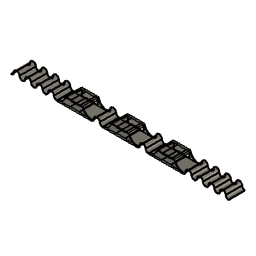
ACUTE_Prototype 4 v1 (Autodesk Fusion 360 design; units mm, degrees)
Autodesk Fusion 360 part; units mm, degrees
note: some values were not read from the file. Chosen so that the rebuilt part matches the saved one: which bodies a step acts on. Set by a fixed rule: which sketch regions a step uses.
sketch "Sketch2" plane through (0, 0, 0) normal (0, 1, 0) x (1, 0, 0)
  line L0 (0, 0) -> (0, -4) construction
  line L1 (0, -4) -> (1, -4) construction
  circle A0 centre (4, -4) radius 4
  circle A1 centre (4, -4) radius 3
  circle A2 centre (11, -4) radius 3
  circle A3 centre (11, -4) radius 4
  circle A4 centre (18, -4) radius 3
  circle A5 centre (18, -4) radius 4
  line L2 (18, 0) -> (18, -1)
  line L3 (18, 0) -> (39, 0)
  line L4 (39, 0) -> (39, -10)
  line L5 (39, -10) -> (18, -10) construction
  line L6 (18, -10) -> (18, 0) construction
  line L7 (28.5, 0) -> (28.5, -10) construction
  line L8 (18, -1) -> (28.5, -1) construction
  arc A6 (28.5, -10) -> (18, -1) centre (18, -11.625) ccw
  line L9 (28.5, -10) -> (39, -10)
  line L10 (4, 0) -> (4, -4)
  line L11 (28.5, 0) -> (29.5, 0) construction
  line L12 (29.5, 0) -> (29.5, -10)
  line L13 (29.5, -10) -> (28.5, -10) construction
  line L14 (28.5, -10) -> (28.5, 0) construction
  line L15 (28.5, -1) -> (29.5, -1) construction
  line L16 (28.5, -1) -> (29.5, -1) construction
  line L17 (29.5, -1) -> (29.5, -1.5) construction
  line L18 (29.5, -1.5) -> (28.5, -1.5) construction
  line L19 (28.5, -1.5) -> (28.5, -1) construction
  line L20 (29.5, -1) -> (39, -1) construction
  line L21 (39, -1) -> (39, -1.4931) construction
  line L22 (39, -1.4931) -> (29.5, -1.4931) construction
  line L23 (29.5, -1.4931) -> (29.5, -1) construction
  line L24 (29.5, -10) -> (39, -10) construction
  line L25 (39, -10) -> (39, -8) construction
  line L26 (39, -8) -> (29.5, -8) construction
  line L27 (29.5, -8) -> (29.5, -10) construction
  line L28 (29.5, -8) -> (39, -8) construction
  line L29 (39, -8) -> (39, -7.5) construction
  line L30 (39, -7.5) -> (29.5, -7.5) construction
  line L31 (29.5, -7.5) -> (29.5, -8) construction
  line L32 (29.5, -8) -> (33.5, -8)
  line L33 (33.5, -8) -> (33.5, -7.5)
  line L34 (33.5, -7.5) -> (29.5, -7.5) construction
  line L35 (29.5, -7.5) -> (29.5, -8) construction
  line L36 (29.5, -1.4931) -> (33.5, -1.4931) construction
  line L37 (33.5, -1.4931) -> (33.5, -0.9931)
  line L38 (33.5, -0.9931) -> (29.5, -0.9931)
  line L39 (29.5, -0.9931) -> (29.5, -1.4931) construction
  line L40 (33.5, -1.4931) -> (39, -1.4931)
  line L41 (39, -1.4931) -> (39, -1) construction
  line L42 (39, -1) -> (33.5, -1) construction
  line L43 (33.5, -1) -> (33.5, -1.4931) construction
  line L44 (33.5, -7.5) -> (39, -7.5)
  line L45 (0, 0) -> (4, 0) construction
  dimension "d1" = 4
  dimension "d2" = 1
  dimension "d3" = 8
  dimension "d4" = 6
  dimension "d7" = 7
  dimension "d8" = 0
  dimension "d13" = 21
  dimension "d14" = 10
  dimension "d17" = 1
  dimension "d18" = 0.5
  dimension "d19" = 2
  dimension "d20" = 0.5
  dimension "d21" = 4
  dimension "d22" = 4
  constraint coincident L0.start L45.start
  constraint vertical L0
  constraint perpendicular L0 L1
  constraint coincident L0.end A0
  constraint coincident L1.end A1
  constraint coincident A0.centre A1.centre
  constraint coincident A5 L2.start
  constraint coincident A4 L2.end
  constraint vertical L2
  constraint horizontal L3
  constraint vertical L4
  constraint horizontal L5
  constraint vertical L6
  constraint coincident A4.centre L6
  constraint midpoint L3 L7.start
  constraint perpendicular L5 L7
  constraint coincident L7 L8.end
  constraint tangent A4 L8
  constraint midpoint L5 L7.end
  constraint tangent L8 A6
  constraint coincident A0 L10.start
  constraint horizontal L11
  constraint vertical L12
  constraint horizontal L13
  constraint vertical L14
  constraint coincident L12 L15.end
  constraint perpendicular L12 L15
  constraint horizontal L16
  constraint vertical L17
  constraint horizontal L18
  constraint vertical L19
  constraint horizontal L20
  constraint vertical L21
  constraint horizontal L22
  constraint vertical L23
  constraint coincident L4 L21.end
  constraint horizontal L24
  constraint vertical L25
  constraint horizontal L26
  constraint vertical L27
  constraint horizontal L28
  constraint vertical L29
  constraint horizontal L30
  constraint vertical L31
  constraint horizontal L32
  constraint vertical L33
  constraint horizontal L34
  constraint vertical L35
  constraint horizontal L36
  constraint vertical L37
  constraint horizontal L38
  constraint vertical L39
  constraint horizontal L40
  constraint vertical L41
  constraint horizontal L42
  constraint vertical L43
  constraint perpendicular L29 L44
  constraint tangent A0 L45
  measures "d1" distance of L0.start L0.end
  measures "d2" distance of L0.end L1.end
  measures "d3" diameter of A0
  measures "d4" diameter of A1
  measures "d13" distance of L2.start L3.end
  measures "d14" distance of L2.start L5.end
  measures "d17" distance of L7.start L11.end
  measures "d18" distance of L8.end L18.end
  measures "d19" distance of L12.end L26.end
  measures "d20" distance of L26.end L30.end
  measures "d21" distance of L26.end L32.end
  measures "d22" distance of L22.end L36.end
extrude "Extrude1" add sketch "Sketch2" along normal blind 20 contours A0 A3 | A0 A2 A3 A5 | A0 A1 A3 L10 | A3 A5 | A3 A4 A5 L2 picked at (14.0564, -6.013) picked at (7.0785, -2.0192) makes body 1
extrude "Extrude5" add sketch "Sketch2" along normal up to surface (20 mm away) separate body contours A5 L3 A6 L9 L12 | A5 L2 A6 | L3 L4 L12 L37 L38 L40 | L4 L9 L12 L32 L33 L44 makes body 2
mirror "Mirror1" about plane through (39, 0, 7.5) normal (1, 0, 0) of bodies 2 merged
sketch "Sketch4" plane through (0, 0, 0) normal (0, -1, 0) x (1, 0, 0)
  arc A0 (15, 4) -> (18, 1) centre (18, 4) ccw
  arc A1 (15, 4) -> (7, 4) centre (11, 4) ccw
  arc A2 (4, 1) -> (7, 4) centre (4, 4) ccw
  line L0 (4, 1) -> (4, 0)
  arc A3 (4, 0) -> (8, 4) centre (4, 4) ccw
  arc A4 (14, 4) -> (8, 4) centre (11, 4) ccw
  arc A5 (14, 4) -> (18, 0) centre (18, 4) ccw
  line L1 (18, 0) -> (18, 1)
  line L2 (44.5, 1.4931) -> (33.5, 1.4931)
  line L3 (33.5, 1.4931) -> (33.5, 0.9931)
  line L4 (33.5, 0.9931) -> (29.5, 0.9931)
  line L5 (29.5, 0.9931) -> (29.5, 8)
  line L6 (29.5, 8) -> (33.5, 8)
  line L7 (33.5, 8) -> (33.5, 7.5)
  line L8 (33.5, 7.5) -> (44.5, 7.5)
  line L9 (44.5, 7.5) -> (44.5, 8)
  line L10 (44.5, 8) -> (48.5, 8)
  line L11 (48.5, 8) -> (48.5, 0.9931)
  line L12 (48.5, 0.9931) -> (44.5, 0.9931)
  line L13 (44.5, 0.9931) -> (44.5, 1.4931)
  line L14 (18, 0) -> (60, 0)
  line L15 (60, 0) -> (60, 1)
  arc A6 (49.5, 10) -> (60, 1) centre (60, 11.625) ccw
  line L16 (49.5, 10) -> (28.5, 10)
  arc A7 (18, 1) -> (28.5, 10) centre (18, 11.625) ccw
  line L17 (18, 1) -> (18, 0)
extrude "Extrude2" add sketch "Sketch4" against normal blind 1 contours L2 L3 L4 L5 L6 L7 L8 L9 L10 L11 L12 L13 bodies 2
sketch "Sketch5" plane through (29.5, 0, 0) normal (1, 0, 0) x (0, 1, 0)
  line L0 (1, 8) -> (1, 0.9931)
  line L1 (1, 0.9931) -> (20, 0.9931)
  line L2 (20, 0.9931) -> (20, 8)
  line L3 (20, 8) -> (1, 8)
  line L4 (20, 8) -> (19, 8)
  line L5 (19, 8) -> (19, 0.9931)
  line L6 (19, 0.9931) -> (20, 0.9931)
  line L7 (20, 0.9931) -> (20, 8)
  line L8 (1, 8) -> (1, 0.9931)
  line L9 (1, 0.9931) -> (20, 0.9931)
  line L10 (20, 0.9931) -> (20, 8)
  line L11 (20, 8) -> (1, 8)
  dimension "d27" = 1
  constraint horizontal L4
  constraint vertical L5
  constraint horizontal L6
  constraint vertical L7
  constraint coincident L2.end L3.start
  measures "d27" distance of L2.end L4.end
extrude "Extrude3" cut sketch "Sketch5" against normal blind 11.5 contours L0 L1 L3 L5 L8 L9 L11 bodies 2
sketch "Sketch6" plane through (48.5, 0, 0) normal (-1, 0, 0) x (0, -1, 0)
  line L0 (-1, 0.9931) -> (-1, 8)
  line L1 (-1, 8) -> (-20, 8)
  line L2 (-20, 8) -> (-20, 0.9931)
  line L3 (-20, 0.9931) -> (-1, 0.9931)
  line L4 (-20, 8) -> (-19, 8)
  line L5 (-19, 8) -> (-19, 0.9931)
  line L6 (-19, 0.9931) -> (-20, 0.9931)
  line L7 (-20, 0.9931) -> (-20, 8)
  line L8 (-1, 0.9931) -> (-1, 8)
  line L9 (-1, 8) -> (-20, 8)
  line L10 (-20, 8) -> (-20, 0.9931)
  line L11 (-20, 0.9931) -> (-1, 0.9931)
  dimension "d30" = 1
  constraint horizontal L4
  constraint vertical L5
  constraint horizontal L6
  constraint vertical L7
  constraint coincident L1.end L2.start
  measures "d30" distance of L1.end L4.end
extrude "Extrude4" cut sketch "Sketch6" against normal blind 11.5 contours L0 L1 L3 L5 L8 L9 L11 bodies 1 2
pattern_linear "R-Pattern1" count 3 spacing 56 along (1, 0, 0) of bodies 1 2 makes body 3 at (64.0037, 13.3333, 4.1495) makes body 4 at (120.0037, 13.3333, 4.1495) makes body 5 at (88, 6.6667, 0) makes body 6 at (144, 6.6667, 0)
combine "Combine1" operation add target body 2 tool bodies 3 4 5 6
ref_plane "WorkPlane1" through (95, 0, 0) normal (1, 0, 0) x (0, 1, 0)
mirror "Mirror2" about plane through (95, 0, 0) normal (1, 0, 0) of bodies 1 makes body 7
pattern_linear "R-Pattern2" count 4 spacing 14 along (-1, 0, 0) of bodies 1 makes body 8 at (-5.9963, 13.3333, 4.1495) makes body 9 at (-19.9963, 13.3333, 4.1495) makes body 10 at (-33.9963, 13.3333, 4.1495)
combine "Combine2" operation add target body 10 tool bodies 9 8
mirror "Mirror3" about plane through (95, 0, 0) normal (1, 0, 0) of bodies 10 makes body 11
combine "Combine3" operation add target body 7 tool bodies 11 2 1 10
equation "d1 = d3 / 2"
equation "d2 = Belt_Thickness"
equation "d3 = Wave_Lenght + Belt_Thickness"
equation "d4 = Wave_Lenght - Belt_Thickness"
equation "d7 = Wave_Lenght"
equation "Length_between_actuators = 21 mm" comment "Number divisible by 7"
equation "Wave_Lenght = Length_between_actuators * 1 / 3"
equation "d35 = Wave_Lenght * 4 + ( 42 * 2 ) * 1 mm"
equation "Belt_Thickness = 1 mm"
equation "d40 = ( Wave_Lenght + Belt_Thickness ) / 2 + ( Wave_Lenght * 2 ) * 2 + 42 mm + ( 42 / 2 ) * 1 mm"
equation "d43 = Num_waves / 2"
equation "d45 = -Wave_Lenght * 2"
equation "Arm_Circumference = 300 mm"
equation "Length_band = Arm_Circumference - ( ( ( 42 * 3 ) * 1 mm ) + ( Wave_Lenght * 8 ) )"
equation "Num_waves = floor(Length_band / ( Wave_Lenght * 2 ))"
